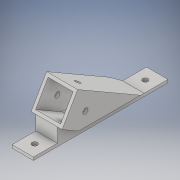
# Autodesk Inventor part: 30DegreeAttachementV04
Saved by Autodesk Inventor 2019.3 (Build 233278000, 278)
## iProperties
Created: 2019-02-16
Part Number: 30DegreeAttachementV04
Material: Generic
Document SubType Name: Modeling
Designer: steele
Density: 1 g/cm^3
Appearance: Default
Author: steele
Autodesk Inventor part; units mm, degrees
note: some values were not read from the file. Chosen so that the rebuilt part matches the saved one: direction of "Hole2".
ref_plane "YZ Plane" through (0, 0, 0) normal (1, 0, 0) x (0, 1, 0)
ref_plane "XZ Plane" through (0, 0, 0) normal (0, 1, 0) x (-1, 0, 0)
ref_plane "XY Plane" through (0, 0, 0) normal (0, 0, 1) x (1, 0, 0)
sketch "Sketch1" plane through (0, 0, 0) normal (1, 0, 0) x (0, 1, 0)
  line L0 (0, 0) -> (15.2005, 26.3281)
  line L1 (15.2005, 26.3281) -> (43.7967, 9.8181)
  line L2 (0, -98.8011) -> (0, 41.6267) projected
  line L3 (43.7967, 9.8181) -> (0, -66.04)
  line L4 (0, 0) -> (0, -66.04)
  line L5 (19.05, 24.1056) -> (0, -8.89) construction
  dimension "d0" = 33.02
  dimension "d1" = 30
  dimension "d5" = 4.445
  dimension "d6" = 38.1
  constraints: 10 end point, 3 point on line, 2 parallel, 1 collinear, 1 perpendicular
  measures "d0" distance of L0.end L1.end
  measures "d1" angle of L0 L2
  measures "d5" distance between parallel lines of L5 L0
  measures "d6" distance from line of L5.end L1
extrude "Extrusion1" add sketch "Sketch1" along normal mid plane 33.02
sketch "Sketch2" plane through (-16.51, 15.2005, 26.3281) normal (0, 0.5, 0.8660254) x (1, 0, 0)
  line L0 (0, 0) -> (33.02, 0) construction
  line L1 (33.02, 0) -> (33.02, 33.02) construction
  line L2 (0, 0) -> (33.02, 33.02) construction
  line L3 (33.02, 33.02) -> (0, 33.02) construction
  line L4 (0, 33.02) -> (33.02, 0) construction
  line L5 (3.175, 3.175) -> (29.845, 3.175)
  line L6 (29.845, 3.175) -> (29.845, 29.845)
  line L7 (29.845, 29.845) -> (3.175, 29.845)
  line L8 (3.175, 29.845) -> (3.175, 3.175)
  line L9 (3.175, 3.175) -> (29.845, 29.845) construction
  line L10 (29.845, 3.175) -> (3.175, 29.845) construction
  point P0 (16.51, 0)
  point P1 (16.51, 16.51)
  dimension "d7" = 26.67
  constraints: 16 end point, 3 midpoint, 2 parallel, 2 perpendicular, 1 horizontal
  measures "d7" distance of L7.end L5.start
extrude "Extrusion2" cut sketch "Sketch2" against normal blind 38.1
sketch "Sketch3" plane through (0, 0, 0) normal (1, 0, 0) x (0, 1, 0)
  line L0 (15.2005, 26.3281) -> (0, 0) projected
  line L1 (0, 0) -> (0, -66.04) projected
  line L2 (0, -66.04) -> (43.7967, 9.8181) projected
  line L3 (21.997, -21.59) -> (0, -8.89) projected
  line L4 (17.9501, 24.7406) -> (0, -6.35) projected
  line L5 (0, 0) -> (0, -66.04)
  line L6 (15.2005, 26.3281) -> (1.6498, 26.3281) construction
  line L7 (0, 0) -> (15.2005, 26.3281) projected
  line L8 (0, 0) -> (0, 51.7281)
  line L9 (43.7967, 9.8181) -> (0, -66.04) projected
  line L10 (0, -66.04) -> (0, -91.44)
  line L11 (0, -134.3611) -> (0, 77.1867) projected
  line L12 (0, 51.7281) -> (-3.175, 51.7281)
  line L13 (-3.175, 51.7281) -> (-3.175, -91.44)
  line L14 (-3.175, -91.44) -> (0, -91.44)
  point P0 (1.0999, -13.335)
  point P1 (0, -15.24)
  point P2 (0, -6.35)
  dimension "d10" = 25.4
  dimension "d11" = 25.4
  dimension "d12" = 3.175
  dimension "supportBaseLength" = 143.1681
  constraints: 14 end point, 5 vertical, 2 horizontal, 2 perpendicular, 3 other
  measures "d10" distance from line of L8.end L6
  measures "d11" distance of L1.end L10.end
  measures "d12" distance of L8.end L12.end
  measures "supportBaseLength" distance between parallel lines of L14 L12
extrude "Extrusion3" add sketch "Sketch3" along normal mid plane 22.86
sketch "Sketch5" plane through (0, 0, 0) normal (1, 0, 0) x (0, 1, 0)
  line L0 (0, 0) -> (15.2005, 26.3281) projected
  line L1 (0, 51.7281) -> (0, 0) projected
  line L2 (15.2005, 26.3281) -> (43.7967, 9.8181) projected
  line L3 (15.2005, 26.3281) -> (0, 26.3281)
  line L4 (0, 0) -> (15.2005, 26.3281)
  constraints: 4 end point, 1 horizontal, 1 point on line
extrude "Extrusion5" add sketch "Sketch5" along normal mid plane 22.86
sketch "Sketch4" plane through (0, 0, 0) normal (0, 0, 1) x (1, 0, 0)
  line L0 (16.51, 43.7967) -> (-16.51, 43.7967) projected
  line L1 (16.51, 0) -> (16.51, 43.7967) projected
  line L2 (16.51, 0) -> (11.43, 0) projected
  line L3 (11.43, 0) -> (-11.43, 0) projected
  line L4 (-11.43, 0) -> (-16.51, 0) projected
  line L5 (-16.51, 43.7967) -> (-16.51, 0) projected
  line L6 (-11.43, 0) -> (-11.43, -3.175) projected
  line L7 (11.43, -3.175) -> (-11.43, -3.175) projected
  line L8 (11.43, -3.175) -> (11.43, 0) projected
  line L9 (-11.43, 0) -> (-16.51, 5.08)
  line L10 (-16.51, 43.7967) -> (-16.51, 0) projected
  line L11 (-16.51, 5.08) -> (-16.51, 0)
  line L12 (0, 0) -> (0, 43.7967) construction
  line L13 (11.43, 0) -> (16.51, 0)
  line L14 (11.43, 0) -> (16.51, 5.08)
  line L15 (16.51, 5.08) -> (16.51, 0)
  dimension "d15" = 45
  constraints: 12 end point, 1 collinear, 1 midpoint, 1 point on line, 1 symmetric about line
  measures "d15" angle of L9 L4
extrude "Extrusion4" cut sketch "Sketch4" against normal up to surface (143.1681 mm away) from surface at 51.7281 contours L1 L2 L14 | L9 L4 L5
sketch "Sketch6" plane through (-11.43, 0, 51.7281) normal (0, 1, 0) x (1, 0, 0)
  line L0 (22.86, 143.1681) -> (0, 143.1681) construction
  line L1 (11.43, 143.1681) -> (11.43, 0) construction
  line L2 (22.86, 0) -> (0, 0) construction
  point P0 (11.43, 51.7281)
  point P1 (11.43, 130.4681)
  point P2 (11.43, 12.7)
  dimension "d21" = 12.7
  dimension "d22" = 12.7
  constraints: 2 end point, 2 midpoint, 2 point on line
  measures "d21" distance from line of point (11.43, 12.7) L2
  measures "d22" distance from line of point (11.43, 130.468) L0
hole "Hole1" at (0, 0, -78.74) at (0, 0, 39.0281) direction (0, -1, 0) diameter 5.6134 end through all clearance for "Flat Head Machine Screw (82)" size "#10" standard "Ansi Unified Screw Threads"
sketch "Sketch9" plane through (0, 0, 0) normal (1, 0, 0) x (0, 1, 0)
  line L0 (1.905, -3.0504) -> (1.905, -9.9899) projected
  line L1 (1.905, -9.9899) -> (21.997, -21.59) projected
  line L2 (41.047, 11.4056) -> (21.997, -21.59) projected
  line L3 (17.9501, 24.7406) -> (41.047, 11.4056) projected
  line L4 (17.9501, 24.7406) -> (1.905, -3.0504) projected
  line L5 (29.4986, 18.0731) -> (10.4486, -14.9225) construction
  line L6 (1.905, -9.9899) -> (21.997, -21.59) construction
  circle A0 centre (19.9736, 1.5753) radius 2.8067
  point P0 (0, 0)
  dimension "d30" = 5.6134
  constraints: 2 end point, 2 midpoint, 1 centre point, 1 perpendicular, 1 point on line
  measures "d30" diameter of A0
extrude "Extrusion6" cut sketch "Sketch9" along normal through all both and the other way through all contours A0
sketch "Sketch10" plane through (-16.51, 43.7967, 9.8181) normal (0, 0.8660254, -0.5) x (1, 0, 0)
  line L0 (3.175, 0) -> (29.845, 0) construction
  line L1 (16.51, 0) -> (16.51, 77.7875) construction
  point P0 (16.51, 30.401)
  point P1 (16.51, 19.05)
  dimension "d33" = 19.05
  constraints: 2 end point, 1 midpoint, 1 point on line, 1 vertical
  measures "d33" distance from line of point (16.51, 19.05) L0
hole "Hole2" at (0, 34.2717, -6.6797) direction (0, -0.8660254, 0.5) diameter 5.6134 depth 3.175 clearance for "Flat Head Machine Screw (82)" size "#10" standard "Ansi Unified Screw Threads"
equation "\"d0\" = widthToSupportExtrusion"
equation "\"d1\" = attachementAngle"
equation "\"d6\" = insertDepth"
equation "\"d2\" = widthToSupportExtrusion"
equation "\"d7\" = insertForExtrusion"
equation "\"d8\" = insertDepth"
equation "\"d12\" = supportBaseDepth"
equation "\"d13\" = supportBaseWidth"
equation "\"attachementAngle\" = 30deg"
equation "\"extrusionSize\" = 25.4"
equation "\"wallThickness\" = 3.175"
equation "\"slipClearance\" = 0.635"
equation "\"insertForExtrusion\" = extrusionSize + 2 * slipClearance"
equation "\"widthToSupportExtrusion\" = insertForExtrusion + 2 * wallThickness"
equation "\"insertDepth\" = 38.1"
equation "\"supportBaseWidth\" = 22.86"
equation "\"supportBaseDepth\" = 3.175"
body "Solid1"
